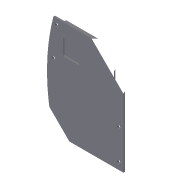
# Autodesk Inventor part: 00_Backplate
Saved by Autodesk Inventor 2016 (Build 200138000, 138)
## iProperties
Created: 2017-04-20
Part Number: 00_Backplate
Material: Generisch
Document SubType Name: Modeling
Designer: diederichbenedict
Density: 1 g/cm^3
Appearance: Vorgabe
Mass: 4.87069 g
Surface Area: 64.6776 cm^2
Volume: 4.87069 cm^3
Author: diederichbenedict
Autodesk Inventor part; units mm, degrees
ref_plane "YZ Plane" through (0, 0, 0) normal (1, 0, 0) x (0, 1, 0)
ref_plane "XZ Plane" through (0, 0, 0) normal (0, 1, 0) x (-1, 0, 0)
ref_plane "XY Plane" through (0, 0, 0) normal (0, 0, 1) x (1, 0, 0)
sketch "Skizze1" plane through (0, 0, 0) normal (0, 1, 0) x (-1, 0, 0)
  line L0 (0, 0) -> (48, 0)
  line L1 (48, 0) -> (48, -63) construction
  line L2 (48, -63) -> (0, -63)
  line L3 (0, -63) -> (0, 0)
  arc A0 (44, -63) -> (44, 0) centre (-78.0312, -31.5) ccw
  line L4 (44, 0) -> (44, -63) construction
  line L5 (44, 0) -> (107, 0) construction
  dimension "d0" = 48
  dimension "d1" = 63
  dimension "d2" = 90
  constraints: 12 end point, 2 horizontal, 2 parallel, 2 perpendicular, 2 point on circle, 2 point on line, 1 centre point
  measures "d0" distance of L1.end L2.end
  measures "d1" distance of L0.end L1.end
  measures "d2" angle of L4 L5
extrude "Extrusion1" add sketch "Skizze1" along normal blind 1
sketch "Skizze2" plane through (0, 1, 0) normal (0, 1, 0) x (1, 0, 0)
  line L0 (-44, 0) -> (0, 0) projected
  line L1 (0, 0) -> (0, 63) projected
  line L2 (0, 63) -> (-44, 63) projected
  arc A0 (-44, 63) -> (-44, 0) centre (78.0312, 31.5) ccw projected
  circle A1 centre (-42, 3.5) radius 1
  circle A2 centre (-2.5, 1.5) radius 1
  circle A3 centre (-44, 22.5) radius 1
  circle A4 centre (-42, 60.5) radius 1
  circle A5 centre (-3, 58.5) radius 1
  circle A6 centre (-3, 39.5) radius 1
  line L3 (-38, 8.5) -> (-28, 8.5)
  line L4 (-28, 8.5) -> (-28, 18.5)
  line L5 (-28, 18.5) -> (-38, 18.5)
  line L6 (-38, 18.5) -> (-38, 8.5)
  point P0 (0, 0)
  dimension "d5" = 2
  dimension "d6" = 3.5
  dimension "d7" = 2
  dimension "d8" = 2
  dimension "d9" = 2
  dimension "d10" = 39.5
  dimension "d11" = 2
  dimension "d12" = 2
  dimension "d13" = 19
  dimension "d14" = 2
  dimension "d15" = 57
  dimension "d16" = 2
  dimension "d17" = 2
  dimension "d18" = 39
  dimension "d19" = 2
  dimension "d20" = 19
  dimension "d21" = 10
  dimension "d22" = 10
  dimension "d23" = 5
  dimension "d24" = 4
  constraints: 8 end point, 6 centre point, 2 parallel, 1 horizontal, 1 perpendicular
  measures "d5" diameter of A1
  measures "d6" distance from line of A1.centre L0
  measures "d7" horizontal distance of A1.centre L0.start
  measures "d8" diameter of A2
  measures "d9" vertical distance of A2.centre A1.centre
  measures "d10" horizontal distance of A2.centre A1.centre
  measures "d11" diameter of A3
  measures "d12" horizontal distance of A1.centre A3.centre
  measures "d13" vertical distance of A1.centre A3.centre
  measures "d14" diameter of A4
  measures "d15" distance of A1.centre A4.centre
  measures "d16" diameter of A5
  measures "d17" vertical distance of A5.centre A4.centre
  measures "d18" horizontal distance of A5.centre A4.centre
  measures "d19" diameter of A6
  measures "d20" distance of A6.centre A5.centre
  measures "d21" distance of L5.end L4.end
  measures "d22" distance of L4.end L3.end
  measures "d23" distance from line of L3 A1.centre
  measures "d24" distance from line of A1.centre L6
extrude "Extrusion2" cut sketch "Skizze2" against normal through all contours A1 | A2 | A3 | A4 | A5 | A6 | L6 L5 L4 L3
sketch "Skizze3" plane through (0, 1, 0) normal (0, 1, 0) x (1, 0, 0)
  circle A0 centre (-3, 39.5) radius 1 projected
  circle A1 centre (-42, 60.5) radius 1 projected
  circle A2 centre (-2.5, 1.5) radius 1 projected
  circle A3 centre (-42, 3.5) radius 1 projected
  circle A4 centre (-44, 22.5) radius 1 projected
  circle A5 centre (-3, 58.5) radius 1 projected
  line L0 (-28, 18.5) -> (-28, 8.5) projected
  line L1 (-28, 8.5) -> (-38, 8.5) projected
  line L2 (-38, 8.5) -> (-38, 18.5) projected
  line L3 (-38, 18.5) -> (-28, 18.5) projected
  line L4 (-44, 0) -> (0, 0) projected
  line L5 (0, 0) -> (0, 63) projected
  line L6 (0, 63) -> (-44, 63) projected
  arc A6 (-44, 63) -> (-44, 0) centre (78.0312, 31.5) ccw projected
  line L7 (-28, 8.5) -> (-38, 8.5) projected
  line L8 (-38, 8.5) -> (-28, 8.5)
  line L9 (-28, 8.5) -> (-28, 18.5)
  line L10 (-28, 18.5) -> (-38, 18.5)
  line L11 (-38, 18.5) -> (-38, 8.5)
  line L12 (-38, 0) -> (-7, 0)
  line L13 (-7, 0) -> (-7, 41)
  line L14 (-7, 41) -> (-38, 41)
  line L15 (-38, 41) -> (-38, 0)
  line L16 (-7, 41) -> (-34, 41)
  line L17 (-34, 41) -> (-34, 55)
  line L18 (-34, 55) -> (-7, 55)
  line L19 (-7, 55) -> (-7, 41)
  point P0 (0, 0)
  dimension "d27" = 31
  dimension "d28" = 41
  dimension "d31" = 27
  dimension "d32" = 8
  constraints: 24 end point, 6 parallel, 3 horizontal, 3 perpendicular, 1 point on line
  measures "d27" distance of L14.end L13.end
  measures "d28" distance of L13.end L12.end
  measures "d31" distance of L17.end L18.end
  measures "d32" distance between parallel lines of L18 L6
extrude "Extrusion3" add sketch "Skizze3" along normal blind 1 contours L3 L15 L14 L13 L4 L1 L0 | L0 L1 L2 L3 | L17 L18 L19 L14
sketch "Skizze4" plane through (0, 2, 0) normal (0, 1, 0) x (1, 0, 0)
  line L0 (-38, 18.5) -> (-28, 18.5) projected
  line L1 (-28, 18.5) -> (-28, 8.5) projected
  line L2 (-28, 8.5) -> (-38, 8.5) projected
  line L3 (-38, 8.5) -> (-38, 18.5) projected
  point P0 (0, 0)
extrude "Extrusion4" add sketch "Skizze4" along normal blind 4
